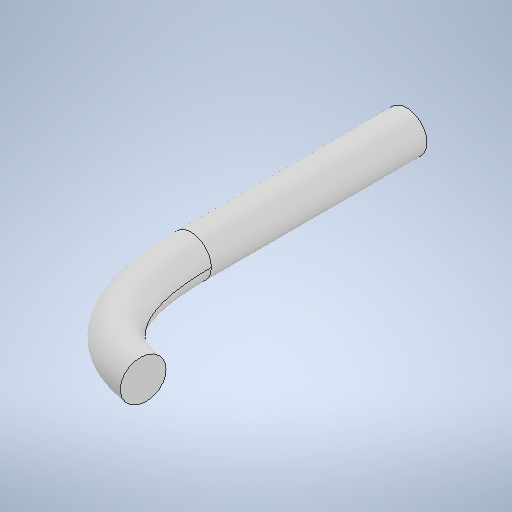
# Autodesk Inventor part: shaft_sweep_vertical
Saved by Autodesk Inventor 2025 (Build 290162000, 162)
## iProperties
Created: 2024-07-12
Part Number: shaft_sweep_vertical
Material: 일반
Document SubType Name: Modeling
Designer: unney
Density: 1 g/cm^3
Appearance: 기본값
Author: unney
Autodesk Inventor part; units mm, degrees
ref_plane "YZ Plane" through (0, 0, 0) normal (1, 0, 0) x (0, 1, 0)
ref_plane "XZ Plane" through (0, 0, 0) normal (0, 1, 0) x (-1, 0, 0)
ref_plane "XY Plane" through (0, 0, 0) normal (0, 0, 1) x (1, 0, 0)
sketch "스케치1" plane through (0, 0, 0) normal (0, 0, 1) x (1, 0, 0)
  circle A0 centre (0, 0) radius 8.5
  dimension "d0" = 17
  constraints: 1 centre point, 1 coincident
  measures "d0" diameter of A0
sketch "스케치4" plane through (0, 0, 0) normal (0, 1, 0) x (-1, 0, 0)
  line L0 (0, 0) -> (0, 90)
  line L1 (0, 90) -> (0, 140) construction
  line L2 (0, 140) -> (-34.7868, 144.7491) construction
  spline S0 degree 2 poles (0, 90) (0, 140) (-34.7868, 144.7491) knots 1 1 1 2 2 2
  dimension "d4" = 90
  dimension "d5" = 50
  constraints: 2 end point, 2 vertical, 3 other
  measures "d4" distance of L0.start L0.end
  measures "d5" distance of L0.end L1.end
sweep "스윕1" add profiles "스케치1" path "스케치4"
